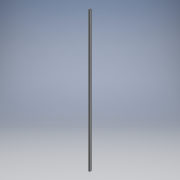
# Autodesk Inventor part: HFS5-4060-4000
Saved by Autodesk Inventor 2019.4 (Build 234330000, 330)
## iProperties
Category: PARTsolutions
Company: MISUMI
Part Number: HFS5-4060-4000
Material: Generic
Catalog Web Link: www.cadenas.de
Description: HFS5-2060, HFS5-2080, HFS5-4060, HFS5-4080, NFS5-2060, NFS5-2080, NFS5-4060, NFS5-4080-HFS5 Series Aluminum Extrusions 20mm Square -3 or more slots-
Vendor: MISUMI
Document SubType Name: Modeling
Designer: partserver
Manufacturer: MISUMI
Mass: 2657.73 g
Surface Area: 27102.5 cm^2
Volume: 2657.73 cm^3
Density: 1 g/cm^3
Appearance: PSOLRGB-175-175-175
PSOL_IDENT_0: {$CADENAS_DATA\23d-libs\misumi\metric\38_al_extrusions_blackets\5\hfs5_2060.prj},624 {VTYP=3D},{NB=H
PSOL_IDENT_1: FS5-4060-4000},{LINA=HFS5-4060-4000},{NN=HFS5-2060, HFS5-2080, HFS5-4060, HFS5-4080, NFS5-2060, NFS5
PSOL_IDENT_2: -2080, NFS5-4060, NFS5-4080},{DATE=09.09.2019 15:28:27},{GEOMDATE=24.05.2018 01:50:00},{VERSION=},{L
PSOL_IDENT_3: INEID=240},{WBVAR=L,ALT1,ALT2,ALT4,ALT5,CP5,DL5,DR5,ALT6,ALT9,ALT10,ALT11,HP6,NHL6,DL6,NHR6,DR6,ALT7
PSOL_IDENT_4: ,ALT8,NH9,AH,BH,CH,DH,EH,NH10,AV,BV,CV,DV,EV,NH11,AP,BP,CP,DP,EP,ALT12,ALT13,Z,NH12,XA,XB,XC,XD,XE,N
PSOL_IDENT_5: H13,YA,YB,YC,YD,YE,ALT16,HP16,DL16,DR16,ALT17,HQ17,JLP,ALT18,HQ18,KLP,ALT20},{WBNUMERIC=L,NH9,AH,BH,
PSOL_IDENT_6: CH,DH,EH,NH10,AV,BV,CV,DV,EV,NH11,AP,BP,CP,DP,EP,NH12,XA,XB,XC,XD,XE,NH13,YA,YB,YC,YD,YE,HQ17,JLP,HQ
PSOL_IDENT_7: 18,KLP}  {NB=HFS5-4060-4000},{LINA=HFS5-4060-4000},{KT=DUMMY},{PN=HFS5-4060-4000},{TPS=HFS5-4060},{M
PSOL_IDENT_8: AT=A6N01SS-T5 Aluminum Alloy},{ST=Clear Anodize},{FRMW=40},{FRMH=60},{FRD=4.2},{L=4000},{MASS=1.80},
PSOL_IDENT_9: {SA=665},{LX=12.63x10^4},{LY=27.0x10^4},{ALT1=},{M1=0},{DPL1=0},{DPR1=0},{ALT1PN=},{ALT2=},{ALT2ALG=
PSOL_IDENT_10: '','w/o End Tapping (Heli-Coil Insert)','LHP','with LHP (Tapping on the Left (Heli-Coil Insert))','
PSOL_IDENT_11: RHP','with RHP (Tapping on the Right (Heli-Coil Insert))','HPW','with HPW (Tapping on Both Ends (Hel
PSOL_IDENT_12: i-Coil Insert))' },{M2=0},{DP2=0},{ALT2PN=},{ALT4=},{ALT4ALG= '', 'Not applicable' },{ALT4PN=},{ALT5=
PSOL_IDENT_13: },{ALT5ALG= '','w/o 45 Degree Cut','1','with 45 Degree Cut' },{CP5=},{CP5ALG= '','N/A' },{DL5=},{DL5
PSOL_IDENT_14: ALG= '','N/A' },{DR5=},{DR5ALG= '','N/A' },{FRMLALT5=0},{FRMRALT5=0},{ALT5PN=},{ALT6=},{ALT6ALG= '','
PSOL_IDENT_15: w/o Fastening Location Wrench Access Hole Alterations','1','with Fastening Location Wrench Access Ho
PSOL_IDENT_16: le Alterations' },{ALT9=},{ALT9ALG= '','w/o Location Specified Wrench Access Hole Alteratons (Horizo
PSOL_IDENT_17: ntal)','1','with Location Specified Wrench Access Hole Alteratons (Horizontal)' },{ALT10=},{ALT10ALG=
PSOL_IDENT_18: '','w/o Location Specified Wrench Access Hole Alteratons (Vertical)','1','with Location Specified W
PSOL_IDENT_19: rench Access Hole Alteratons (Vertical)' },{ALT11=},{ALT11ALG= '','w/o Location Specified Wrench Acc
PSOL_IDENT_20: ess Hole Alteratons (Crisscross)','1','with Location Specified Wrench Access Hole Alteratons (Crissc
PSOL_IDENT_21: ross)' },{DD6=0.00},{DD6ALG=0},{HP6=},{HP6ALG= '','N/A' },{NHL6=},{NHL6ALG= '','N/A' },{DL6=},{DL6AL
PSOL_IDENT_22: G= '','N/A' },{NHR6=},{NHR6ALG= '','N/A' },{DR6=},{DR6ALG= '','N/A' },{DD6PN=},{HL6=0},{HL6D=0},{HR6=
PSOL_IDENT_23: 0},{HR6D=0},{J6=0},{J6D=0},{K6=0},{K6D=0},{ALT7=},{ALT7ALG= '','N/A' },{ALT8=},{ALT8ALG= '','N/A' },
PSOL_IDENT_24: {ALT678PN=},{NH9=0},{NH9MAX=5},{NH9ALG=[0]},{AH=0.0},{AHMIN=7},{AHMAX=3995},{AHALG=[0]},{BH=0.0},{BH
PSOL_IDENT_25: MIN=2},{BHMAX=3997},{BHALG=[0]},{CH=0.0},{CHMIN=2},{CHMAX=3999},{CHALG=[0]},{DH=0.0},{DHMIN=2},{DHMA
PSOL_IDENT_26: X=4001},{DHALG=[0]},{EH=0.0},{EHMIN=2},{EHMAX=3993},{EHALG=[0]},{NH10=0},{NH10MAX=5},{NH10ALG=[0]},{
PSOL_IDENT_27: AV=0.0},{AVMIN=7},{AVMAX=3995},{AVALG=[0]},{BV=0.0},{BVMIN=2},{BVMAX=3997},{BVALG=[0]},{CV=0.0},{CVM
PSOL_IDENT_28: IN=2},{CVMAX=3999},{CVALG=[0]},{DV=0.0},{DVMIN=2},{DVMAX=4001},{DVALG=[0]},{EV=0.0},{EVMIN=2},{EVMAX=
PSOL_IDENT_29: 3993},{EVALG=[0]},{NH11=0},{NH11MAX=5},{NH11ALG=[0]},{AP=0.0},{APMIN=7},{APMAX=3995},{APALG=[0]},{BP=
PSOL_IDENT_30: 0.0},{BPMIN=2},{BPMAX=3997},{BPALG=[0]},{CP=0.0},{CPMIN=2},{CPMAX=3999},{CPALG=[0]},{DP=0.0},{DPMIN=
PSOL_IDENT_31: 2},{DPMAX=4001},{DPALG=[0]},{EP=0.0},{EPMIN=2},{EPMAX=3993},{EPALG=[0]},{ALT9PN=},{ALT10PN=},{ALT11P
PSOL_IDENT_32: N=},{ALT91011PN=},{ALT12=},{ALT12ALG= '','w/o Counterbore Hole in Specified Position (Vertical)','1'
PSOL_IDENT_33: ,'with Counterbore Hole in Specified Position (Vertical)' },{ALT13=},{ALT13ALG= '','w/o Counterbore
PSOL_IDENT_34: Hole in Specified Position (Horizontal)','1','with Counterbore Hole in Specified Position (Horizonta
PSOL_IDENT_35: l)' },{Z=},{ZALG= '','N/A' },{DD12=0.0},{DD112=0.0},{NH12=0},{NH12MAX=5},{NH12ALG=[0]},{XA=0.0},{XAM
PSOL_IDENT_36: IN=7},{XAMAX=3995},{XAALG=[0]},{XB=0.0},{XBMIN=2},{XBMAX=3997},{XBALG=[0]},{XC=0.0},{XCMIN=2},{XCMAX=
PSOL_IDENT_37: 3999},{XCALG=[0]},{XD=0.0},{XDMIN=2},{XDMAX=4001},{XDALG=[0]},{XE=0.0},{XEMIN=2},{XEMAX=3993},{XEALG=
PSOL_IDENT_38: [0]},{NH13=0},{NH13MAX=5},{NH13ALG=[0]},{YA=0.0},{YAMIN=7},{YAMAX=3995},{YAALG=[0]},{YB=0.0},{YBMIN=
PSOL_IDENT_39: 2},{YBMAX=3997},{YBALG=[0]},{YC=0.0},{YCMIN=2},{YCMAX=3999},{YCALG=[0]},{YD=0.0},{YDMIN=2},{YDMAX=40
PSOL_IDENT_40: 01},{YDALG=[0]},{YE=0.0},{YEMIN=2},{YEMAX=3993},{YEALG=[0]},{ALT12PN=},{ALT13PN=},{ALT1213PN=},{ALT1
PSOL_IDENT_41: 6=},{ALT16ALG= '','w/o M Type Hole Alteration','1','with M Type Hole Alteration' },{HP16=},{HP16ALG=
PSOL_IDENT_42: '','N/A' },{DL16=},{DL16ALG= '','N/A' },{DR16=},{DR16ALG= '','N/A' },{H116=0},{D16=0.0},{ALT16PN=},
PSOL_IDENT_43: {ALT17=},{ALT17ALG= '','w/o L Type Hole Alteration (Top)','1','with L Type Hole Alteration (Top)' },
PSOL_IDENT_44: {HQ17=0},{HQ17ALG=0},{JLP=0},{JLPMIN=4.9},{JLPMAX=0},{JLPALG=[0]},{L17=0},{D17=0.0},{ALT17PN=},{ALT1
PSOL_IDENT_45: 8=},{ALT18ALG= '','w/o L Type Hole Alteration (Bottom)','1','with L Type Hole Alteration (Bottom)' }
PSOL_IDENT_46: ,{HQ18=0},{HQ18ALG=0},{KLP=0},{KLPMIN=4.9},{KLPMAX=0},{KLPALG=[0]},{L18=0},{D18=0.0},{ALT18PN=},{ALT
PSOL_IDENT_47: 20=},{ALT20PN=},{ERRORALT01=OK},{ERRORALT02=OK},{ERRORALT05=OK},{ERRORALT06091=OK},{ERRORALT06092=OK
PSOL_IDENT_48: },{ERRORALT06093=OK},{ERRORALT06094=OK},{ERRORALT06101=OK},{ERRORALT06102=OK},{ERRORALT06103=OK},{ER
PSOL_IDENT_49: RORALT06104=OK},{ERRORALT06111=OK},{ERRORALT06112=OK},{ERRORALT06113=OK},{ERRORALT06114=OK},{ERRORAL
PSOL_IDENT_50: T06121=OK},{ERRORALT06122=OK},{ERRORALT06123=OK},{ERRORALT06124=OK},{ERRORALT06131=OK},{ERRORALT0613
PSOL_IDENT_51: 2=OK},{ERRORALT06133=OK},{ERRORALT06134=OK},{ERRORALT0616=OK},{ERRORALT06171=OK},{ERRORALT06172=OK},
PSOL_IDENT_52: {ERRORALT06173=OK},{ERRORALT06181=OK},{ERRORALT06182=OK},{ERRORALT06183=OK},{ERRORALT0911=OK},{ERROR
PSOL_IDENT_53: ALT0913=OK},{ERRORALT0916=OK},{ERRORALT0917=OK},{ERRORALT0918=OK},{ERRORALT1011=OK},{ERRORALT1012=OK
PSOL_IDENT_54: },{ERRORALT1016=OK},{ERRORALT1017=OK},{ERRORALT1018=OK},{ERRORALT1112=OK},{ERRORALT1113=OK},{ERRORAL
PSOL_IDENT_55: T1116=OK},{ERRORALT1117=OK},{ERRORALT1118=OK},{ERRORALT1216=OK},{ERRORALT1217=OK},{ERRORALT1218=OK},
PSOL_IDENT_56: {ERRORALT1316=OK},{ERRORALT1317=OK},{ERRORALT1318=OK},{ERRORALT1617=OK},{ERRORALT1618=OK},{ERRORPN=}
PSOL_IDENT_57: ,{TFW=0}
NB: HFS5-4060-4000
NN: HFS5-2060, HFS5-2080, HFS5-4060, HFS5-4080, NFS5-2060, NFS5-2080, NFS5-4060, NFS5-4080
NT: HFS5 Series Aluminum Extrusions 20mm Square -3 or more slots-
NBSYN: $PN.
LINA: HFS5-4060-4000
CATALOG: Misumi
PN: HFS5-4060-4000
TPS: HFS5-4060
MAT: A6N01SS-T5 Aluminum Alloy
ST: Clear Anodize
L: 4000
MASS: 1.80
SA: 665
LX: 12.63x10^4
LY: 27.0x10^4
ALT1: w/o End Tapping
M1: 0
DPL1: 0
DPR1: 0
ALT2: w/o End Tapping (Heli-Coil Insert)
M2: 0
DP2: 0
ALT4: Not applicable
ALT5: w/o 45 Degree Cut
CP5: N/A
DL5: N/A
DR5: N/A
ALT6: w/o Fastening Location Wrench Access Hole Alterations
ALT9: w/o Location Specified Wrench Access Hole Alteratons (Horizontal)
ALT10: w/o Location Specified Wrench Access Hole Alteratons (Vertical)
ALT11: w/o Location Specified Wrench Access Hole Alteratons (Crisscross)
DD6: 0
HP6: N/A
NHL6: N/A
DL6: N/A
NHR6: N/A
DR6: N/A
HL6D: 0
HR6D: 0
J6D: 0
K6D: 0
ALT7: N/A
ALT8: N/A
NH9: 0
AH: 0
BH: 0
CH: 0
DH: 0
EH: 0
NH10: 0
AV: 0
BV: 0
CV: 0
DV: 0
EV: 0
NH11: 0
AP: 0
BP: 0
CP: 0
DP: 0
EP: 0
ALT12: w/o Counterbore Hole in Specified Position (Vertical)
ALT13: w/o Counterbore Hole in Specified Position (Horizontal)
Z: N/A
DD12: 0
DD112: 0
NH12: 0
XA: 0
XB: 0
XC: 0
XD: 0
XE: 0
NH13: 0
YA: 0
YB: 0
YC: 0
YD: 0
YE: 0
ALT16: w/o M Type Hole Alteration
HP16: N/A
DL16: N/A
DR16: N/A
H116: 0
D16: 0
ALT17: w/o L Type Hole Alteration (Top)
HQ17: 0
JLP: 0
D17: 0
ALT18: w/o L Type Hole Alteration (Bottom)
HQ18: 0
KLP: 0
D18: 0
ALT20: w/o CW (End Face C Chamfering)
SUPPLIER: MISUMI
ARTICLENO: HFS5-4060-4000
BOMINFO: HFS5-4060-4000
CREATOR: CADENAS GmbH
Title: HFS5-4060-4000
Author: Cadenas PARTsolutions
Comments: HFS5 Series Aluminum Extrusions 20mm Square -3 or more slots-
Autodesk Inventor part; units mm, degrees
ref_plane "YZ Plane" through (0, 0, 0) normal (1, 0, 0) x (0, 1, 0)
ref_plane "XZ Plane" through (0, 0, 0) normal (0, 1, 0) x (-1, 0, 0)
ref_plane "XY Plane" through (0, 0, 0) normal (0, 0, 1) x (1, 0, 0)
sketch "Sketch_100" plane through (0, 0, 0) normal (0, 0, 1) x (1, 0, 0)
  line L0 (-20, -3) -> (-20, -17)
  line L1 (-20, -17) -> (-18, -17)
  line L2 (-18, -17) -> (-18, -14)
  line L3 (-18, -14) -> (-17.0607, -14)
  line L4 (-17.0607, -14) -> (-14, -17.0607)
  line L5 (-14, -17.0607) -> (-14, -19.4804)
  line L6 (-14, -19.4804) -> (-13.7, -20)
  line L7 (-13.7, -20) -> (-14, -20.5196)
  line L8 (-14, -20.5196) -> (-14, -22.9393)
  line L9 (-14, -22.9393) -> (-17.0607, -26)
  line L10 (-17.0607, -26) -> (-18, -26)
  line L11 (-18, -26) -> (-18, -23)
  line L12 (-18, -23) -> (-20, -23)
  line L13 (-20, -23) -> (-20, -29)
  arc A0 (-20, -29) -> (-19, -30) centre (-19, -29) ccw
  line L14 (-19, -30) -> (-13, -30)
  line L15 (-13, -30) -> (-13, -28)
  line L16 (-13, -28) -> (-16, -28)
  line L17 (-16, -28) -> (-16, -27.0607)
  line L18 (-16, -27.0607) -> (-12.9393, -24)
  line L19 (-12.9393, -24) -> (-10.5196, -24)
  line L20 (-10.5196, -24) -> (-10, -23.7)
  line L21 (-10, -23.7) -> (-9.4804, -24)
  line L22 (-9.4804, -24) -> (-7.0607, -24)
  line L23 (-7.0607, -24) -> (-4, -27.0607)
  line L24 (-4, -27.0607) -> (-4, -28)
  line L25 (-4, -28) -> (-7, -28)
  line L26 (-7, -28) -> (-7, -30)
  line L27 (-7, -30) -> (7, -30)
  line L28 (7, -30) -> (7, -28)
  line L29 (7, -28) -> (4, -28)
  line L30 (4, -28) -> (4, -27.0607)
  line L31 (4, -27.0607) -> (7.0607, -24)
  line L32 (7.0607, -24) -> (9.4804, -24)
  line L33 (9.4804, -24) -> (10, -23.7)
  line L34 (10, -23.7) -> (10.5196, -24)
  line L35 (10.5196, -24) -> (12.9393, -24)
  line L36 (12.9393, -24) -> (16, -27.0607)
  line L37 (16, -27.0607) -> (16, -28)
  line L38 (16, -28) -> (13, -28)
  line L39 (13, -28) -> (13, -30)
  line L40 (13, -30) -> (19, -30)
  arc A1 (19, -30) -> (20, -29) centre (19, -29) ccw
  line L41 (20, -29) -> (20, -23)
  line L42 (20, -23) -> (18, -23)
  line L43 (18, -23) -> (18, -26)
  line L44 (18, -26) -> (17.0607, -26)
  line L45 (17.0607, -26) -> (14, -22.9393)
  line L46 (14, -22.9393) -> (14, -20.5196)
  line L47 (14, -20.5196) -> (13.7, -20)
  line L48 (13.7, -20) -> (14, -19.4804)
  line L49 (14, -19.4804) -> (14, -17.0607)
  line L50 (14, -17.0607) -> (17.0607, -14)
  line L51 (17.0607, -14) -> (18, -14)
  line L52 (18, -14) -> (18, -17)
  line L53 (18, -17) -> (20, -17)
  line L54 (20, -17) -> (20, -3)
  line L55 (20, -3) -> (18, -3)
  line L56 (18, -3) -> (18, -6)
  line L57 (18, -6) -> (17.0607, -6)
  line L58 (17.0607, -6) -> (14, -2.9393)
  line L59 (14, -2.9393) -> (14, -0.5196)
  line L60 (14, -0.5196) -> (13.7, 0)
  line L61 (13.7, 0) -> (14, 0.5196)
  line L62 (14, 0.5196) -> (14, 2.9393)
  line L63 (14, 2.9393) -> (17.0607, 6)
  line L64 (17.0607, 6) -> (18, 6)
  line L65 (18, 6) -> (18, 3)
  line L66 (18, 3) -> (20, 3)
  line L67 (20, 3) -> (20, 17)
  line L68 (20, 17) -> (18, 17)
  line L69 (18, 17) -> (18, 14)
  line L70 (18, 14) -> (17.0607, 14)
  line L71 (17.0607, 14) -> (14, 17.0607)
  line L72 (14, 17.0607) -> (14, 19.4804)
  line L73 (14, 19.4804) -> (13.7, 20)
  line L74 (13.7, 20) -> (14, 20.5196)
  line L75 (14, 20.5196) -> (14, 22.9393)
  line L76 (14, 22.9393) -> (17.0607, 26)
  line L77 (17.0607, 26) -> (18, 26)
  line L78 (18, 26) -> (18, 23)
  line L79 (18, 23) -> (20, 23)
  line L80 (20, 23) -> (20, 29)
  arc A2 (20, 29) -> (19, 30) centre (19, 29) ccw
  line L81 (19, 30) -> (13, 30)
  line L82 (13, 30) -> (13, 28)
  line L83 (13, 28) -> (16, 28)
  line L84 (16, 28) -> (16, 27.0607)
  line L85 (16, 27.0607) -> (12.9393, 24)
  line L86 (12.9393, 24) -> (10.5196, 24)
  line L87 (10.5196, 24) -> (10, 23.7)
  line L88 (10, 23.7) -> (9.4804, 24)
  line L89 (9.4804, 24) -> (7.0607, 24)
  line L90 (7.0607, 24) -> (4, 27.0607)
  line L91 (4, 27.0607) -> (4, 28)
  line L92 (4, 28) -> (7, 28)
  line L93 (7, 28) -> (7, 30)
  line L94 (7, 30) -> (-7, 30)
  line L95 (-7, 30) -> (-7, 28)
  line L96 (-7, 28) -> (-4, 28)
  line L97 (-4, 28) -> (-4, 27.0607)
  line L98 (-4, 27.0607) -> (-7.0607, 24)
  line L99 (-7.0607, 24) -> (-9.4804, 24)
  line L100 (-9.4804, 24) -> (-10, 23.7)
  line L101 (-10, 23.7) -> (-10.5196, 24)
  line L102 (-10.5196, 24) -> (-12.9393, 24)
  line L103 (-12.9393, 24) -> (-16, 27.0607)
  line L104 (-16, 27.0607) -> (-16, 28)
  line L105 (-16, 28) -> (-13, 28)
  line L106 (-13, 28) -> (-13, 30)
  line L107 (-13, 30) -> (-19, 30)
  arc A3 (-19, 30) -> (-20, 29) centre (-19, 29) ccw
  line L108 (-20, 29) -> (-20, 23)
  line L109 (-20, 23) -> (-18, 23)
  line L110 (-18, 23) -> (-18, 26)
  line L111 (-18, 26) -> (-17.0607, 26)
  line L112 (-17.0607, 26) -> (-14, 22.9393)
  line L113 (-14, 22.9393) -> (-14, 20.5196)
  line L114 (-14, 20.5196) -> (-13.7, 20)
  line L115 (-13.7, 20) -> (-14, 19.4804)
  line L116 (-14, 19.4804) -> (-14, 17.0607)
  line L117 (-14, 17.0607) -> (-17.0607, 14)
  line L118 (-17.0607, 14) -> (-18, 14)
  line L119 (-18, 14) -> (-18, 17)
  line L120 (-18, 17) -> (-20, 17)
  line L121 (-20, 17) -> (-20, 3)
  line L122 (-20, 3) -> (-18, 3)
  line L123 (-18, 3) -> (-18, 6)
  line L124 (-18, 6) -> (-17.0607, 6)
  line L125 (-17.0607, 6) -> (-14, 2.9393)
  line L126 (-14, 2.9393) -> (-14, 0.5196)
  line L127 (-14, 0.5196) -> (-13.7, 0)
  line L128 (-13.7, 0) -> (-14, -0.5196)
  line L129 (-14, -0.5196) -> (-14, -2.9393)
  line L130 (-14, -2.9393) -> (-17.0607, -6)
  line L131 (-17.0607, -6) -> (-18, -6)
  line L132 (-18, -6) -> (-18, -3)
  line L133 (-18, -3) -> (-20, -3)
  line L134 (-18, 8) -> (-16.9393, 8)
  line L135 (-16.9393, 8) -> (-12.5, 3.5607)
  line L136 (-12.5, 3.5607) -> (-12.5, 0.75)
  line L137 (-12.5, 0.75) -> (12.5, 0.75)
  line L138 (12.5, 0.75) -> (12.5, 3.5607)
  line L139 (12.5, 3.5607) -> (16.9393, 8)
  line L140 (16.9393, 8) -> (18, 8)
  line L141 (18, 8) -> (18, 12)
  line L142 (18, 12) -> (16.9393, 12)
  line L143 (16.9393, 12) -> (12.9393, 16)
  line L144 (12.9393, 16) -> (8, 16)
  arc A4 (6, 18) -> (8, 16) centre (8, 18) ccw
  line L145 (6, 18) -> (6, 22.9393)
  line L146 (6, 22.9393) -> (2, 26.9393)
  line L147 (2, 26.9393) -> (2, 28)
  line L148 (2, 28) -> (-2, 28)
  line L149 (-2, 28) -> (-2, 26.9393)
  line L150 (-2, 26.9393) -> (-6, 22.9393)
  line L151 (-6, 22.9393) -> (-6, 18)
  arc A5 (-8, 16) -> (-6, 18) centre (-8, 18) ccw
  line L152 (-8, 16) -> (-12.9393, 16)
  line L153 (-12.9393, 16) -> (-16.9393, 12)
  line L154 (-16.9393, 12) -> (-18, 12)
  line L155 (-18, 12) -> (-18, 8)
  line L156 (-18, -8) -> (-18, -12)
  line L157 (-18, -12) -> (-16.9393, -12)
  line L158 (-16.9393, -12) -> (-12.9393, -16)
  line L159 (-12.9393, -16) -> (-8, -16)
  arc A6 (-6, -18) -> (-8, -16) centre (-8, -18) ccw
  line L160 (-6, -18) -> (-6, -22.9393)
  line L161 (-6, -22.9393) -> (-2, -26.9393)
  line L162 (-2, -26.9393) -> (-2, -28)
  line L163 (-2, -28) -> (2, -28)
  line L164 (2, -28) -> (2, -26.9393)
  line L165 (2, -26.9393) -> (6, -22.9393)
  line L166 (6, -22.9393) -> (6, -18)
  arc A7 (8, -16) -> (6, -18) centre (8, -18) ccw
  line L167 (8, -16) -> (12.9393, -16)
  line L168 (12.9393, -16) -> (16.9393, -12)
  line L169 (16.9393, -12) -> (18, -12)
  line L170 (18, -12) -> (18, -8)
  line L171 (18, -8) -> (16.9393, -8)
  line L172 (16.9393, -8) -> (12.5, -3.5607)
  line L173 (12.5, -3.5607) -> (12.5, -0.75)
  line L174 (12.5, -0.75) -> (-12.5, -0.75)
  line L175 (-12.5, -0.75) -> (-12.5, -3.5607)
  line L176 (-12.5, -3.5607) -> (-16.9393, -8)
  line L177 (-16.9393, -8) -> (-18, -8)
  constraints: 356 end point, 16 point on circle, 8 centre point
extrude "Extrusion1" add sketch "Sketch_100" against normal blind 4000
sketch "Sketch2" plane through (0, 0, 0) normal (0, 0, 1) x (1, 0, 0)
  point P0 (10, 20)
hole "Hole1" at (10, 20, 0) direction (0, 0, -1) diameter 4.2 depth 4000
pattern_linear "Rectangular Pattern1" count 2 spacing 20 along (-1, 0, 0) count 2 spacing 40 along (0, -1, 0) of "Hole1"
move faces "Move1" translate (0, 0, 2725) faces at (-4.1667, 0.25, -4000)
move faces "Move2" translate (0, 0, -2725) faces at (-4.1667, 0.25, -1275)
body "Solid1"
